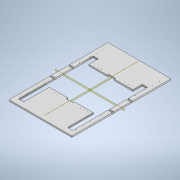
# Autodesk Inventor part: top_part
Saved by Autodesk Inventor 2020 (Build 240168000, 168)
## iProperties
Created: 2019-12-27
Part Number: top_part
Material: Générique
Document SubType Name: Modeling
Designer: damien
Density: 1 g/cm^3
Appearance: Par défaut
Author: damien
Autodesk Inventor part; units mm, degrees
ref_plane "YZ Plane" through (0, 0, 0) normal (1, 0, 0) x (0, 1, 0)
ref_plane "XZ Plane" through (0, 0, 0) normal (0, 1, 0) x (-1, 0, 0)
ref_plane "XY Plane" through (0, 0, 0) normal (0, 0, 1) x (1, 0, 0)
sketch "Esquisse1" plane through (0, 0, 0) normal (0, 1, 0) x (-1, 0, 0)
  line L0 (-460, -725) -> (460, -725)
  line L1 (460, -725) -> (460, 725)
  line L2 (460, 725) -> (-460, 725)
  line L3 (-460, 725) -> (-460, -725)
  line L4 (-460, -725) -> (460, 725) construction
  line L5 (460, -725) -> (-460, 725) construction
  point P0 (0, 0)
  dimension "d0" = 1450
  dimension "d1" = 920
  constraints: 12 end point, 2 midpoint, 2 parallel, 1 horizontal, 1 perpendicular
  measures "d0" distance of L0.end L1.end
  measures "d1" distance of L1.end L2.end
extrude "Extrusion1" add sketch "Esquisse1" along normal blind 21
sketch "Esquisse2" plane through (0, 21, 0) normal (0, 1, 0) x (1, 0, 0)
  line L0 (-398, -649) -> (-398, 444)
  line L1 (-398, 444) -> (-323, 444)
  line L2 (-323, 444) -> (-323, 307)
  line L3 (-323, 307) -> (323, 307)
  line L4 (323, 307) -> (323, 444)
  line L5 (323, 444) -> (398, 444)
  line L6 (398, 444) -> (398, -649)
  line L7 (398, -649) -> (323, -649)
  line L8 (323, -649) -> (323, -273)
  line L9 (323, -273) -> (-323, -273)
  line L10 (-323, -273) -> (-323, -649)
  line L11 (-323, -649) -> (-398, -649)
  line L12 (460, -725) -> (460, 725) projected
  line L13 (-460, 725) -> (-460, -725) projected
  line L14 (-460, -725) -> (460, -725) projected
  line L15 (460, 725) -> (-460, 725) projected
  line L16 (-460, 0) -> (-398, 0) construction
  line L17 (460, 0) -> (398, 0) construction
  point P0 (0, 0)
  dimension "d4" = 1093
  dimension "d5" = 75
  dimension "d7" = 580
  dimension "d8" = 137
  dimension "d55" = 646
  dimension "d56" = 281
  constraints: 28 end point, 9 point on line, 8 perpendicular, 3 equal length, 2 midpoint, 2 vertical
  measures "d4" distance of L5.end L6.end
  measures "d5" distance of L6.end L7.end
  measures "d7" distance between parallel lines of L3 L9
  measures "d8" distance of L3.end L4.end
  measures "d55" distance between parallel lines of L8 L10
  measures "d56" distance between parallel lines of L15 L1
extrude "Extrusion2" cut sketch "Esquisse2" against normal blind 21.1 contours L0 L1 L2 L3 L4 L5 L6 L7 L8 L9 L10 L11
sketch "Esquisse3" plane through (-460, 0, 575) normal (1, 0, 0) x (0, 0, -1)
  line L0 (-74, 21) -> (1019, 21) projected
  line L1 (438, 21) -> (462, 21)
  line L2 (462, 21) -> (462, 11)
  line L3 (462, 11) -> (438, 11)
  line L4 (438, 11) -> (438, 21)
  line L5 (-150, 0) -> (-150, 21) projected
  line L6 (711, 21) -> (735, 21)
  line L7 (735, 21) -> (735, 11)
  line L8 (735, 11) -> (711, 11)
  line L9 (711, 11) -> (711, 21)
  line L10 (882, 21) -> (882, 0) projected
  line L11 (302, 21) -> (302, 0) projected
  point P0 (575, 0)
  point P1 (462, 21)
  dimension "d14" = 24
  dimension "d15" = 10
  dimension "d17" = 24
  dimension "d57" = 147
  dimension "d58" = 136
  constraints: 16 end point, 4 parallel, 2 horizontal, 2 perpendicular, 2 point on line, 1 collinear
  measures "d14" distance of L2.end L3.end
  measures "d15" distance of L1.end L2.end
  measures "d17" distance of L7.end L8.end
  measures "d57" distance between parallel lines of L10 L7
  measures "d58" distance between parallel lines of L11 L4
extrude "Extrusion3" cut sketch "Esquisse3" along normal blind 1000
sketch "Esquisse4" plane through (0, 21, 0) normal (0, 1, 0) x (1, 0, 0)
  line L0 (323, 307) -> (-323, 307) projected
  line L1 (-50, 307) -> (50, 307)
  line L2 (50, 307) -> (50, 327)
  line L3 (50, 327) -> (-50, 327)
  line L4 (-50, 327) -> (-50, 307)
  line L5 (-323, -273) -> (323, -273) projected
  line L6 (-50, -273) -> (50, -273)
  line L7 (50, -273) -> (50, -296)
  line L8 (50, -296) -> (-50, -296)
  line L9 (-50, -296) -> (-50, -273)
  line L10 (-323, 444) -> (-323, 307) projected
  line L11 (323, 307) -> (323, 444) projected
  point P0 (0, 0)
  point P1 (50, -273)
  point P2 (50, 307)
  point P3 (0, 307)
  dimension "d20" = 23
  dimension "d21" = 100
  dimension "d50" = 20
  constraints: 16 end point, 4 parallel, 4 point on line, 2 horizontal, 2 midpoint, 2 perpendicular
  measures "d20" distance of L6.end L7.end
  measures "d21" distance of L2.end L3.end
  measures "d50" distance of L1.end L2.end
extrude "Extrusion4" cut sketch "Esquisse4" against normal blind 100
fillet "Congé1" radius 2 8 edges at (50, 10.5, -327) (50, 10.5, -307) (-50, 10.5, -327) (-50, 10.5, -307) (-50, 10.5, 273) (-50, 10.5, 296) (50, 10.5, 296) (50, 10.5, 273)
sketch "Esquisse5" plane through (0, 21, 0) normal (0, 1, 0) x (1, 0, 0)
  circle A0 centre (0, 507) radius 2.25
  circle A1 centre (0, 407) radius 2.25
  line L0 (-460, 725) -> (-460, -725) projected
  line L1 (460, -725) -> (460, 725) projected
  circle A2 centre (0, 607) radius 2.25
  line L2 (-323, 307) -> (-52, 307) projected
  circle A3 centre (410, 607) radius 2.25
  circle A4 centre (410, 507) radius 2.25
  circle A5 centre (410, 407) radius 2.25
  circle A6 centre (-408, 407) radius 2.25
  circle A7 centre (-408, 507) radius 2.25
  circle A8 centre (-408, 607) radius 2.25
  circle A9 centre (-408, 257) radius 2.25
  circle A10 centre (410, 257) radius 2.25
  line L3 (0, 407) -> (0, 327) construction
  line L4 (48, 327) -> (-48, 327) projected
  point P0 (0, 0)
  point P1 (-460, 160)
  dimension "d29" = 100
  dimension "d30" = 100
  dimension "d32" = 100
  dimension "d35" = 50
  dimension "d36" = 52
  dimension "d51" = 150
  dimension "d52" = 4.5
  constraints: 11 centre point, 11 equal radius, 8 vertical alignment, 7 horizontal alignment, 2 end point, 1 midpoint, 1 vertical
  measures "d29" distance of A0.centre L3.start
  measures "d30" distance of A0.centre A2.centre
  measures "d32" distance from line of L3.start L2
  measures "d35" distance from line of L1 A4.centre
  measures "d36" distance from line of L0 A6.centre
  measures "d51" distance of A9.centre A6.centre
  measures "d52" diameter of A1
extrude "Extrusion5" cut sketch "Esquisse5" against normal blind 100
mirror "Symétrie1" about plane through (0, 0, 0) normal (0, 0, 1) of "Extrusion5"
sketch "Esquisse6" plane through (0, 21, 0) normal (0, 1, 0) x (1, 0, 0)
  circle A0 centre (-270.5, -305) radius 2.25
  line L0 (-323, -649) -> (-323, -273) projected
  line L1 (-323, -305) -> (323, -305) construction
  line L2 (323, -649) -> (323, -273) projected
  line L3 (48, -296) -> (-48, -296) projected
  circle A1 centre (-220.5, -305) radius 2.25
  circle A2 centre (-170.5, -305) radius 2.25
  line L4 (-48, -296) -> (48, -296) projected
  line L5 (0, -296) -> (0, -725) construction
  line L6 (-460, -725) -> (460, -725) projected
  circle A3 centre (270.5, -305) radius 2.25
  circle A4 centre (220.5, -305) radius 2.25
  circle A5 centre (170.5, -305) radius 2.25
  point P0 (0, 0)
  dimension "d37" = 4.5
  dimension "d38" = 9
  dimension "d39" = 52.5
  dimension "d42" = 50
  constraints: 6 centre point, 4 end point, 3 midpoint, 3 point on line, 3 symmetric about line, 2 horizontal, 1 vertical, 7 other
  measures "d37" diameter of A0
  measures "d38" distance between parallel lines of L1 L3
  measures "d39" distance from line of L0 A0.centre
  measures "d42" distance of A0.centre A1.centre
extrude "Extrusion6" cut sketch "Esquisse6" against normal blind 100
sketch "Esquisse7" plane through (0, 21, 0) normal (0, 1, 0) x (1, 0, 0)
  circle A0 centre (270.5, 339) radius 2.25
  circle A1 centre (220.5, 339) radius 2.25
  circle A2 centre (170.5, 339) radius 2.25
  circle A3 centre (-170.5, 339) radius 2.25
  circle A4 centre (-220.5, 339) radius 2.25
  circle A5 centre (-270.5, 339) radius 2.25
  line L0 (323, 307) -> (323, 444) projected
  circle A6 centre (270.5, -305) radius 2.25 projected
  line L1 (50, 325) -> (50, 309) projected
  circle A7 centre (-270.5, -305) radius 2.25 projected
  line L2 (-52, -273) -> (-323, -273) projected
  line L3 (-323, 307) -> (-52, 307) projected
  point P0 (0, 0)
  dimension "d60" = 50
  dimension "d61" = 50
  dimension "d62" = 120.5
  dimension "d63" = 50
  dimension "d64" = 50
  dimension "d66" = 32
  constraints: 6 centre point, 6 equal radius, 5 horizontal alignment, 2 vertical alignment
  measures "d60" distance of A0.centre A1.centre
  measures "d61" distance of A1.centre A2.centre
  measures "d62" distance from line of A2.centre L1
  measures "d63" distance of A4.centre A5.centre
  measures "d64" distance of A3.centre A4.centre
  measures "d66" distance from line of L3 A5.centre
fillet "Congé2" radius 5 4 edges at (460, 10.5, -725) (-460, 10.5, -725) (-460, 10.5, 725) (460, 10.5, 725)
ref_plane "Plan de construction2" through (0, 21, -136) normal (-1, 0, 0) x (0, 0, 1)
extrude "Extrusion7" cut sketch "Esquisse7" against normal blind 21 contours A0 | A1 | A2 | A3 | A4 | A5
ref_plane "Plan de construction1" through (0, 0, 0) normal (0, 0, 1) x (1, 0, 0)
